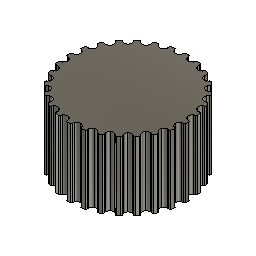
gear_28z (Autodesk Fusion 360 design; units mm, degrees)
Autodesk Fusion 360 part; units mm, degrees
sketch "Sketch1" plane through (0, 0, 0) normal (0, 0, 1) x (1, 0, 0) in component "gt2 pulley"
  circle A0 centre (0, 0) radius 8.9127 construction
  circle A1 centre (0, 0) radius 7.9087 construction
  line L0 (0, 0) -> (0, 8.9127) construction
  line L1 (0, 0) -> (0.9979, 8.8566) construction
  line L2 (0, 0) -> (1.4105, 8.8004) construction
  circle A2 centre (0, 0) radius 8.6587 construction
  arc A3 (0.3711, 8.5115) -> (0.4204, 8.237) centre (1.3703, 8.5496) ccw
  circle A4 centre (0, 0) radius 8.5087 construction
  arc A5 (0.225, 8.6558) -> (0, 8.6587) centre (0, 0) ccw
  arc A6 (0.3711, 8.5115) -> (0.225, 8.6558) centre (0.2212, 8.5058) ccw
  arc A7 (0.4204, 8.237) -> (0.8855, 7.8589) centre (0.9476, 8.4105) ccw
  arc A8 (0, 8.6587) -> (-0.225, 8.6558) centre (0, 0) ccw
  arc A9 (-0.225, 8.6558) -> (-0.3711, 8.5115) centre (-0.2212, 8.5058) ccw
  arc A10 (-0.4204, 8.237) -> (-0.3711, 8.5115) centre (-1.3703, 8.5496) ccw
  arc A11 (-0.8855, 7.8589) -> (-0.4204, 8.237) centre (-0.9476, 8.4105) ccw
  arc A12 (0.8855, 7.8589) -> (-0.8855, 7.8589) centre (0, 0) ccw
  point P0 (1.3703, 8.5496)
  point P1 (0, 8.6587)
  dimension "d18" = 17.8254
  dimension "d19" = 6.429
  dimension "d22" = 1.004
  dimension "d24" = 0.75
  dimension "d26" = 1
  dimension "d27" = 0.15
  dimension "d28" = 0.15
  dimension "d47" = 0.555
  dimension "d52" = 3.812
  constraint coincident A0.centre A1.centre
  constraint coincident A0 L0.end
  constraint vertical L0
  constraint coincident A0 L1.end
  constraint coincident A0 L2.end
  constraint concentric A1 A2
  constraint coincident A1 A7.end
  constraint coincident L1 A7.end
  constraint coincident A2 P0
  constraint coincident L2 P0
  constraint coincident P0 A3.centre
  constraint coincident A2 P1
  constraint coincident L0 P1
  constraint concentric A2 A4
  constraint coincident P1 A5.end
  constraint coincident A4 A6.centre
  constraint coincident A3.start A6.start
  constraint tangent A3 A6
  constraint tangent A3 A7
  constraint symmetric L0 A7.end A11.start
  constraint symmetric L0 A3.start A9.end
  constraint symmetric L0 A3.end A10.start
  constraint symmetric L0 A3 A10
  constraint symmetric L0 A5.start A8.end
  constraint symmetric L0 P1 A5.end
  constraint symmetric L0 A5 A8
  constraint symmetric L0 A6 A9
  constraint symmetric L0 A7 A11
  constraint coincident A1 A11.start
  constraint tangent A1 A7
  constraint coincident L1 A7.centre
  measures "d18" diameter of A0
  measures "d19" angle of L0 L1
  measures "d22" distance of A0 A1
  measures "d24" distance of A1 A2
  measures "d26" radius of A3
  measures "d27" distance of A2 A4
  measures "d28" radius of A6
  measures "d47" radius of A7
extrude "Extrude1" add sketch "Sketch1" along normal blind 10 makes body 1
pattern_circular "C-Pattern1" count 28 over 360 about axis through (0, 0, 1.75) along (0, 0, 1) of bodies 1 makes body 2 at (-1.0811, 7.8344, 6.6667) makes body 3 at (-4.0394, 6.7993, 6.6667) makes body 4 at (-5.4511, 5.73, 6.6667) makes body 5 at (-6.5895, 4.3733, 6.6667) makes body 6 at (-7.1677, 3.3423, 6.6667) makes body 7 at (-7.7317, 1.6636, 6.6667) makes body 8 at (-7.8786, -0.6893, 6.6667) makes body 9 at (-7.5277, -2.4252, 6.6667) makes body 10 at (-6.7993, -4.0394, 6.6667) makes body 11 at (-5.73, -5.4511, 6.6667) makes body 12 at (-4.3733, -6.5895, 6.6667) makes body 13 at (-3.3423, -7.1677, 6.6667) makes body 14 at (-1.6636, -7.7317, 6.6667) makes body 15 at (0.0986, -7.9081, 6.6667) makes body 16 at (1.0811, -7.8344, 6.6667) makes body 17 at (4.0394, -6.7993, 6.6667) makes body 18 at (5.4511, -5.73, 6.6667) makes body 19 at (6.2442, -4.8535, 6.6667) makes body 20 at (7.3974, -2.7974, 6.6667) makes body 21 at (7.8344, -1.0811, 6.6667) makes body 22 at (7.9081, 0.0986, 6.6667) makes body 23 at (7.5277, 2.4252, 6.6667) makes body 24 at (6.7993, 4.0394, 6.6667) makes body 25 at (6.5895, 4.3733, 3.3333) makes body 26 at (4.8535, 6.2442, 6.6667) makes body 27 at (4.0394, 6.7993, 6.6667) makes body 28 at (1.0811, 7.8344, 6.6667)
sketch "Sketch2" plane through (0, 0, 10) normal (0, 0, 1) x (-1, 0, 0)
  arc A0 (-7.8296, -3.3587) -> (-7.8962, -3.5529) centre (-7.7594, -3.4913) ccw
  arc A1 (-7.8962, -3.5529) -> (-7.7009, -3.9583) centre (0, 0) ccw
  arc A2 (-7.7009, -3.9583) -> (-7.5076, -4.0273) centre (-7.5675, -3.8898) ccw
  arc A3 (-7.2388, -3.9527) -> (-7.5076, -4.0273) centre (-7.1083, -4.9441) ccw
  arc A4 (-6.6965, -4.2077) -> (-7.2388, -3.9527) centre (-7.1664, -4.5029) ccw
  arc A5 (-7.4649, -2.6121) -> (-6.6965, -4.2077) centre (0, 0) ccw
  arc A6 (-7.6037, -3.1951) -> (-7.4649, -2.6121) centre (-7.9887, -2.7954) ccw
  arc A7 (-7.8296, -3.3587) -> (-7.6037, -3.1951) centre (-8.2974, -2.4749) ccw
  circle A8 centre (0, 0) radius 7.9087
  constraint concentric A1 A8
extrude "Extrude2" add sketch "Sketch2" against normal blind 10 contours A5 A8 bodies 1 2 3 4 5 6 7 8 9 10 11 12 13 14 15 16 17 18 19 20 21 22 23 24 25 26 27 28
extrude "Extrude4" [suppressed] in component "gt2 pulley"
pattern_circular "C-Pattern7" [suppressed] in component "gt2 pulley"
extrude "Extrude3" [suppressed] in component "gt2 pulley"
pattern_circular "C-Pattern6" [suppressed] in component "gt2 pulley"
extrude "Extrude2'" [suppressed] in component "gt2 pulley"
pattern_circular "C-Pattern5" [suppressed] in component "gt2 pulley"
extrude "Extrude1'" [suppressed] in component "gt2 pulley"
pattern_circular "C-Pattern4" [suppressed] in component "gt2 pulley"
pattern_circular "C-Pattern3" [suppressed] in component "gt2 pulley"
pattern_circular "C-Pattern2" [suppressed] in component "gt2 pulley"
pattern_circular "C-Pattern1'" [suppressed] in component "gt2 pulley"
copy_body "Body->Comp1" [suppressed] in component "Component"
copy_body "Body->Comp2" [suppressed] in component "Component'"
copy_body "Body->Comp3" [suppressed] in component "Component''"
copy_body "Body->Comp4" [suppressed] in component "Component'''"
copy_body "Body->Comp5" [suppressed] in component "Component''''"
copy_body "Body->Comp6" [suppressed] in component "Component'''''"
copy_body "Body->Comp7" [suppressed] in component "Component''''''"
copy_body "Body->Comp8" [suppressed] in component "Component'''''''"
copy_body "Body->Comp9" [suppressed] in component "Component''''''''"
copy_body "Body->Comp10" [suppressed] in component "Component'''''''''"
copy_body "Body->Comp11" [suppressed] in component "Component''''''''''"
copy_body "Body->Comp12" [suppressed] in component "Component'''''''''''"
copy_body "Body->Comp13" [suppressed] in component "Component''''''''''''"
copy_body "Body->Comp14" [suppressed] in component "Component'''''''''''''"
copy_body "Body->Comp15" [suppressed] in component "Component''''''''''''''"
copy_body "Body->Comp16" [suppressed] in component "Component'''''''''''''''"
copy_body "Body->Comp17" [suppressed] in component "Component''''''''''''''''"
copy_body "Body->Comp18" [suppressed] in component "Component'''''''''''''''''"
copy_body "Body->Comp19" [suppressed] in component "Component''''''''''''''''''"
copy_body "Body->Comp20" [suppressed] in component "Component'''''''''''''''''''"
component "gt2 pulley" placed x (1, 0, 0) y (0, 1, 0) z (0, 0, 1) at (0, 0, 0)
equation "NumTeeth = 28" comment "min 20"
equation "ToothPitch = 2 mm"
equation "PullyDia = NumTeeth * ToothPitch / PI"
equation "ToothAng = ( ( 360 / NumTeeth ) * 1 deg )"
equation "TransOffsetAngle = ToothAng * 0.2"
equation "Sholulder_Radius = 0.15 mm"
equation "Root_Radius = 0.555 mm"
equation "TransRadius = 1 mm"
equation "ToolHeight = 0.75 mm"
equation "PLD = 0.254 mm"
equation "d18 = PullyDia"
equation "d19 = ToothAng / 2"
equation "d22 = PLD + ToolHeight"
equation "d24 = ToolHeight"
equation "d26 = TransRadius"
equation "d27 = Sholulder_Radius"
equation "d31 = NumTeeth"
equation "d33 = NumTeeth"
equation "d35 = NumTeeth"
equation "d37 = NumTeeth"
equation "d41 = NumTeeth"
equation "d45 = NumTeeth"
equation "d47 = Root_Radius"
equation "d50 = NumTeeth"
